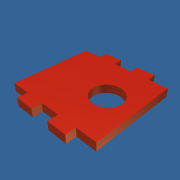
# Autodesk Inventor part: Acrylic_2.2_UpperArmBridge_cameraMount
Saved by Autodesk Inventor 2012 (Build 160160000, 160)
## iProperties
Created: 2014-03-29
Part Number: Acrylic_2.2_UpperArmBridge_cameraMount
Material: Default
Document SubType Name: Modeling
Designer: Admin
Density: 1 g/cm^3
Author: Admin
Autodesk Inventor part; units mm, degrees
ref_plane "YZ Plane" through (0, 0, 0) normal (1, 0, 0) x (0, 1, 0)
ref_plane "XZ Plane" through (0, 0, 0) normal (0, 1, 0) x (-1, 0, 0)
ref_plane "XY Plane" through (0, 0, 0) normal (0, 0, 1) x (1, 0, 0)
sketch "Sketch1" plane through (0, 0, 0) normal (0, 0, 1) x (1, 0, 0)
  line L0 (-19.44, 0) -> (11.99, 0) projected
  line L1 (0, -18.9) -> (0, 18.9) projected
  line L2 (-2.5, -11) -> (-2.5, -13.5)
  line L3 (-2.5, -13.5) -> (2.5, -13.5)
  line L4 (2.5, -13.5) -> (2.5, -11)
  line L5 (-2.5, 11) -> (-2.5, 13.5)
  line L6 (-2.5, 13.5) -> (2.5, 13.5)
  line L7 (2.5, 13.5) -> (2.5, 11)
  line L8 (7.5, 11) -> (7.5, -11)
  line L9 (-7.5, 11) -> (-2.5, 11)
  line L10 (2.5, 11) -> (7.5, 11)
  line L11 (7.5, -11) -> (2.5, -11)
  line L12 (-2.5, -11) -> (-7.5, -11)
  circle A0 centre (0, 0) radius 4
  line L13 (-12.5, 11) -> (-14.95, 11)
  line L14 (-14.95, -11) -> (-12.5, -11)
  line L15 (-7.5, -11) -> (-7.5, -13.5)
  line L16 (-7.5, -13.5) -> (-12.5, -13.5)
  line L17 (-12.5, -13.5) -> (-12.5, -11)
  line L18 (-7.5, 11) -> (-7.5, 13.5)
  line L19 (-7.5, 13.5) -> (-12.5, 13.5)
  line L20 (-12.5, 13.5) -> (-12.5, 11)
  line L21 (-14.95, -11) -> (-14.95, 11)
  circle A1 centre (-10.95, 0) radius 1.5
  dimension "d8" = 2.5
  dimension "d20" = 8
  dimension "d24" = 5
  dimension "d25" = 5
  dimension "d28" = 3
  dimension "d29" = 4
  constraints: 40 end point, 10 perpendicular, 7 parallel, 3 point on line, 2 centre point, 2 horizontal, 1 coincident, 1 vertical
  measures "d8" distance between parallel lines of L4 L1
  measures "d20" diameter of A0
  measures "d24" distance between parallel lines of L2 L15
  measures "d25" distance of L15.end L16.end
  measures "d28" diameter of A1
  measures "d29" distance from line of L21 A1.centre
extrude "Extrusion1" add sketch "Sketch1" along normal blind 2.2 contours L21 L13 L20 L19 L18 L9 L5 L6 L1 A0 L0 A1 | L0 A1 A0 L1 L3 L2 L12 L15 L16 L17 L14 L21 | L1 L6 L7 L10 L8 L0 A0 | A0 L0 L8 L11 L4 L3 L1
equation "\"d2\" = 0.5 * d1"
equation "\"d15\" = 0.5 * d14"
equation "\"d1\" = 50"
equation "\"d14\" = 22"
body "Solid1"
